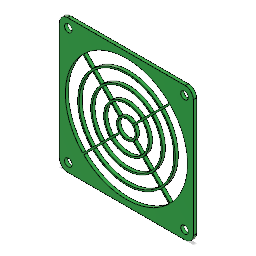
fan guard (Autodesk Fusion 360 design; units mm, degrees)
Autodesk Fusion 360 part; units mm, degrees
sketch "Sketch1" plane through (0, 0, 0) normal (0, 0, 1) x (1, 0, 0)
  circle A0 centre (0, 0) radius 5.75
  circle A1 centre (0, 0) radius 13.6875
  circle A2 centre (0, 0) radius 21.625
  circle A3 centre (0, 0) radius 29.5625
  circle A4 centre (0, 0) radius 37.5
  line L0 (-4.0659, 4.0659) -> (-26.5165, 26.5165)
  line L1 (0, 0) -> (-41.2, 0)
  line L2 (-41.2, 0) -> (-41.2, 36.2)
  line L3 (-36.2, 41.2) -> (0, 41.2)
  line L4 (0, 41.2) -> (0, 0)
  arc A5 (-36.2, 41.2) -> (-41.2, 36.2) centre (-36.2, 36.2) ccw
  line L5 (0, 0) -> (-1.2367, 5.6154) construction
  line L6 (-6.3585, 28.8706) -> (-8.0657, 36.6223) construction
  line L7 (-4.6512, 21.1189) -> (-6.3585, 28.8706) construction
  line L8 (-2.944, 13.3671) -> (-4.6512, 21.1189) construction
  line L9 (-1.2367, 5.6154) -> (-2.944, 13.3671) construction
  circle A6 centre (-35.75, 35.75) radius 2.3
  point P0 (-41.2, 41.2)
  dimension "d140" = 75
  dimension "d141" = 41.2
  dimension "d142" = 41.2
  dimension "d143" = 5
  dimension "d144" = 45
  dimension "d145" = 11.5
  dimension "d146" = 35.75
  dimension "d147" = 35.75
  dimension "d148" = 4.6
  measures "d140" diameter of A4
  measures "d141" distance of L1.end P0
  measures "d142" distance of P0 L3.end
  measures "d143" radius of A5
  measures "d144" angle of L0 L1
  measures "d145" diameter of A0
  measures "d146" distance of L1 A6.centre
  measures "d147" distance of L4 A6.centre
  measures "d148" diameter of A6
extrude "Extrude1" add sketch "Sketch1" along normal blind 2 contours A4 L1 L2 L3 L4 A5 makes body 1
surface "Extrude2" add extruded along (0, 0, 1) between 0 and 2 path "Sketch1" along A1 A0 L0 A2 A3 separate body makes body 2 at (29.5258, -1.4736, 1.3333)
thicken "Thicken1" add thickness 0.5 on both sides 5 faces at (-5.7214, 0.5725, 1.3333) (-13.6195, 1.3628, 1.3333) (-21.5175, 2.1532, 1.3333) (-29.4156, 2.9435, 1.3333) (-19.033, 19.033, 0.6667) on bodies 2 bodies 1
pattern_circular "C-Pattern1" count 4 over 360 about axis through (0, 0, 1.75) along (0, 0, 1) of bodies 1 makes body 7 at (-39.555, -15.2482, 0) makes body 8 at (15.2482, -39.555, 0) makes body 9 at (39.555, 15.2482, 0)
delete_body "RemoveBody1" bodies 2
delete_body "RemoveBody2" bodies 3
delete_body "RemoveBody3" bodies 4
delete_body "RemoveBody4" bodies 5
delete_body "RemoveBody5" bodies 6
combine "Combine1" operation add target body 1 tool bodies 7 8 9
equation "d142 = d141"
equation "d147 = d146"
equation "d148 = m4_hole_diameter"
equation "m4_hole_diameter = 4.6 mm"
